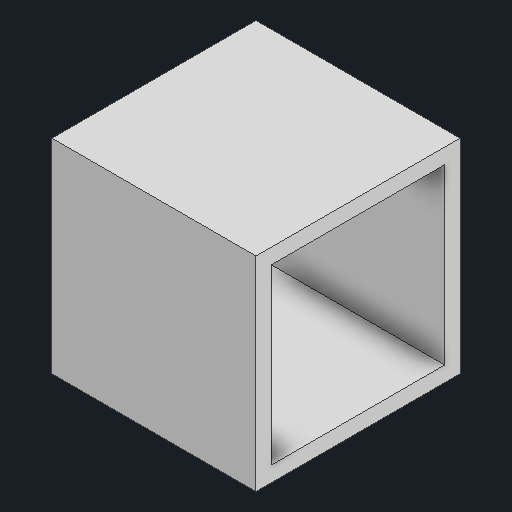
# Autodesk Inventor part: arm
Saved by Autodesk Inventor 2024 (Build 280153000, 153)
## iProperties
Created: 2023-05-03
Part Number: arm
Material: Типовые
Document SubType Name: Modeling
Designer: user
Density: 1 g/cm^3
Appearance: По умолчанию
Author: user
Autodesk Inventor part; units mm, degrees
ref_plane "YZ Plane" through (0, 0, 0) normal (1, 0, 0) x (0, 1, 0)
ref_plane "XZ Plane" through (0, 0, 0) normal (0, 1, 0) x (-1, 0, 0)
ref_plane "XY Plane" through (0, 0, 0) normal (0, 0, 1) x (1, 0, 0)
sketch "Эскиз1" plane through (0, 0, 0) normal (1, 0, 0) x (0, 1, 0)
  line L0 (16.7932, 4.1754) -> (-3.2068, 4.1754) projected
  line L1 (-3.2068, 4.1754) -> (-3.2068, 24.1754)
  line L2 (-3.2068, 24.1754) -> (16.7932, 24.1754)
  line L3 (16.7932, 24.1754) -> (16.7932, 4.1754)
  line L4 (-1.7068, 5.6754) -> (15.2932, 5.6754)
  line L5 (15.2932, 5.6754) -> (15.2932, 22.6754)
  line L6 (15.2932, 22.6754) -> (-1.7068, 22.6754)
  line L7 (-1.7068, 22.6754) -> (-1.7068, 5.6754)
  point P0 (6.7932, 5.6754)
  point P1 (6.7932, 4.1754)
  dimension "d1" = 20
  dimension "d2" = 1.5
  dimension "d3" = 1.5
  constraints: 14 end point, 2 horizontal, 2 midpoint, 2 parallel, 2 perpendicular, 2 vertical, 1 vertical alignment
  measures "d1" distance of L0.end L1.end
  measures "d2" distance from line of L0.end L4
  measures "d3" horizontal distance of L0.end L4.start
extrude "Выдавливание1" add sketch "Эскиз1" against normal blind 20
